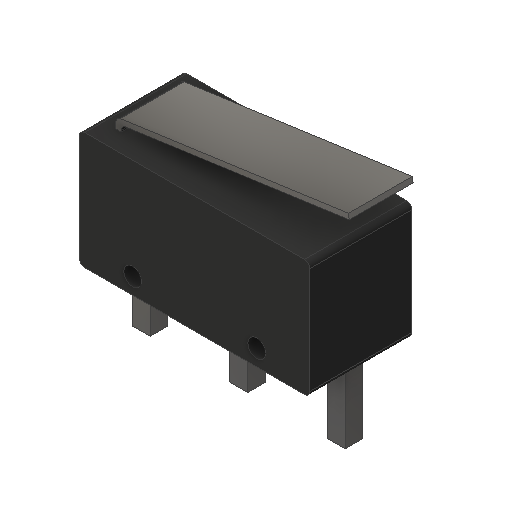
# Autodesk Inventor part: COTS_OMRON_D2FS-FL_Endstop
Saved by Autodesk Inventor 2025 (Build 290162010, 162A)
## iProperties
Created: 2018-07-21
Part Number: COTS_OMRON_D2FS-FL_Endstop
Material: Generic
Document SubType Name: Modeling
Designer: Andrzej
Density: 1 g/cm^3
Appearance: Rubber - Black
Author: Andrzej
Autodesk Inventor part; units mm, degrees
ref_plane "YZ Plane" through (0, 0, 0) normal (1, 0, 0) x (0, 1, 0)
ref_plane "XZ Plane" through (0, 0, 0) normal (0, 1, 0) x (-1, 0, 0)
ref_plane "XY Plane" through (0, 0, 0) normal (0, 0, 1) x (1, 0, 0)
sketch "Sketch1" plane through (0, 0, 0) normal (0, 0, 1) x (1, 0, 0)
  line L0 (-6.5078, 3.6754) -> (6.4922, 3.6754)
  line L1 (6.4922, 3.6754) -> (6.4922, -2.9246)
  line L2 (6.4922, -2.9246) -> (-6.5078, -2.9246)
  line L3 (-6.5078, -2.9246) -> (-6.5078, 3.6754)
  circle A0 centre (-3.5078, -2.0134) radius 0.5
  circle A1 centre (3.4922, -2.0134) radius 0.5
  point P0 (0, 0)
  dimension "d0" = 13
  dimension "d1" = 6.6
  dimension "d2" = 1
  dimension "d3" = 1
  dimension "d4" = 3
  dimension "d5" = 3
  constraints: 8 end point, 2 centre point, 2 parallel, 1 horizontal, 1 horizontal alignment, 1 perpendicular
  measures "d0" distance of L1.end L2.end
  measures "d1" distance of L0.end L1.end
  measures "d2" diameter of A0
  measures "d3" diameter of A1
  measures "d4" distance from line of L3 A0.centre
  measures "d5" distance from line of L1 A1.centre
extrude "Extrusion1" add sketch "Sketch1" along normal blind 5.75
ref_plane "Work Plane1" through (0, 0, 4.7) normal (0, 0, 1) x (1, 0, 0)
sketch "Sketch2" plane through (0, 0, 4.7) normal (0, 0, 1) x (1, 0, 0)
  circle A0 centre (3.4922, -2.0134) radius 0.5 projected
  circle A1 centre (-3.5078, -2.0134) radius 0.5 projected
  line L0 (6.4922, 3.6754) -> (6.4922, -2.9246) projected
  line L1 (6.4922, -2.9246) -> (-6.5078, -2.9246) projected
  line L2 (-6.5078, -2.9246) -> (-6.5078, 3.6754) projected
  line L3 (-6.5078, 3.6754) -> (6.4922, 3.6754) projected
  line L4 (-5.5078, 3.6754) -> (-5.5078, 4.2754)
  line L5 (-5.2078, 3.6754) -> (-5.2078, 4.0146)
  line L6 (-5.2078, 4.0146) -> (7.6657, 5.8238)
  line L7 (-5.2078, 4.0146) -> (7.7922, 4.0146) construction
  line L8 (-5.5078, 4.2754) -> (7.624, 6.1209)
  line L9 (7.624, 6.1209) -> (7.6657, 5.8238)
  point P0 (0, 0)
  dimension "d9" = 0.6
  dimension "d10" = 0.3
  dimension "d11" = 1
  dimension "d12" = 13
  dimension "d13" = 8
  dimension "d14" = 0.3
  constraints: 12 end point, 2 point on line, 2 vertical, 1 equal length, 1 horizontal, 1 perpendicular
  measures "d9" distance of L4.start L4.end
  measures "d10" distance between parallel lines of L5 L4
  measures "d11" distance between parallel lines of L2 L4
  measures "d12" distance of L5.end L6.end
  measures "d13" angle of L7 L6
  measures "d14" distance between parallel lines of L6 L8
extrude "Extrusion2" add sketch "Sketch2" against normal blind 3.6 contours L3 L4 L8 L9 L6 L5
sketch "Sketch3" plane through (-6.5078, -2.9246, 0) normal (0, -1, 0) x (1, 0, 0)
  line L0 (13, 0) -> (0, 0) projected
  line L1 (13, 0) -> (13, 5.75) projected
  line L2 (0, 5.75) -> (13, 5.75) projected
  line L3 (0, 0) -> (0, 5.75) projected
  line L4 (12.5, 2.2589) -> (11.5, 2.2589)
  line L5 (11.5, 2.2589) -> (11.5, 3.2589)
  line L6 (11.5, 3.2589) -> (12.5, 3.2589)
  line L7 (12.5, 3.2589) -> (12.5, 2.2589)
  line L8 (7, 2.2589) -> (6, 2.2589)
  line L9 (6, 2.2589) -> (6, 3.2589)
  line L10 (6, 3.2589) -> (7, 3.2589)
  line L11 (7, 3.2589) -> (7, 2.2589)
  line L12 (1.5, 2.2589) -> (0.5, 2.2589)
  line L13 (0.5, 2.2589) -> (0.5, 3.2589)
  line L14 (0.5, 3.2589) -> (1.5, 3.2589)
  line L15 (1.5, 3.2589) -> (1.5, 2.2589)
  point P0 (6.5078, 0)
  dimension "d17" = 1
  dimension "d18" = 1
  dimension "d19" = 0.5
  dimension "d22" = 5.5
  constraints: 24 end point, 2 horizontal, 2 parallel, 1 perpendicular, 16 other
  measures "d17" distance of L5.end L6.end
  measures "d18" distance of L4.end L5.end
  measures "d19" distance between parallel lines of L1 L7
  measures "d22" distance of L4.start L8.start
extrude "Extrusion3" add sketch "Sketch3" along normal blind 4 contours L4 L5 L6 L7 | L8 L9 L10 L11 | L12 L13 L14 L15
fillet "Fillet1" radius 0.3 4 edges at (6.4922, 3.6754, 2.875) (6.4922, -2.9246, 2.875) (-6.5078, 3.6754, 2.875) (-6.5078, -2.9246, 2.875)
fillet "Fillet2" radius 0.3 2 edges at (-5.5078, 4.2754, 2.9) (-5.2078, 4.0146, 2.9)
equation "\"d5\" = d4"
equation "\"d14\" = d10"
body "Solid1"
